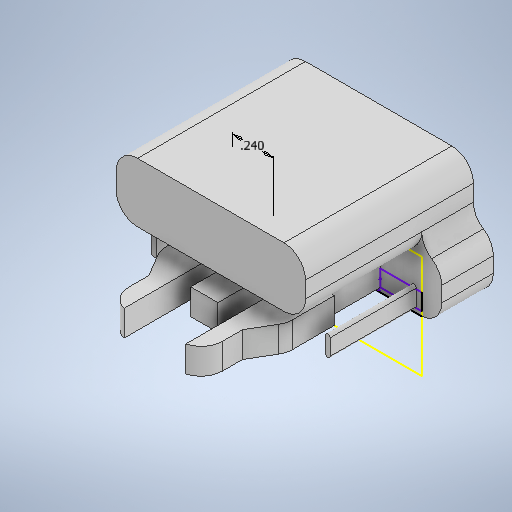
# Autodesk Inventor part: Attachment9
Saved by Autodesk Inventor 2025 (Build 290162010, 162A)
## iProperties
Created: 2026-02-26
Part Number: Attachment9
Material: Generic
Document SubType Name: Modeling
Designer: 925699
Density: 1 g/cm^3
Appearance: Default
Author: 925699
Autodesk Inventor part; units mm, degrees
ref_plane "YZ Plane" through (0, 0, 0) normal (1, 0, 0) x (0, 1, 0)
ref_plane "XZ Plane" through (0, 0, 0) normal (0, 1, 0) x (-1, 0, 0)
ref_plane "XY Plane" through (0, 0, 0) normal (0, 0, 1) x (1, 0, 0)
sketch "Sketch1" plane through (0, 0, 0) normal (0, 0, 1) x (1, 0, 0)
  line L0 (-6.3366, 6.9163) -> (21.6034, 6.9163)
  line L1 (21.6034, 6.9163) -> (21.6034, -8.3237)
  line L2 (21.6034, -8.3237) -> (-6.3366, -8.3237)
  line L3 (-6.3366, -8.3237) -> (-6.3366, 6.9163)
  point P0 (0, 0)
  dimension "d0" = 27.94
  dimension "d1" = 15.24
  constraints: 8 end point, 2 parallel, 1 horizontal, 1 perpendicular
  measures "d0" distance of L1.end L2.end
  measures "d1" distance of L0.end L1.end
extrude "Extrusion1" add sketch "Sketch1" along normal blind 7.62
sketch "Sketch2" plane through (0, 0, 7.62) normal (0, 0, 1) x (1, 0, 0)
  line L0 (-6.3366, 6.9163) -> (-6.3366, -8.3237) projected
  line L1 (21.6034, -8.3237) -> (21.6034, 6.9163) projected
  line L2 (21.6034, -0.052) -> (21.6034, 2.361)
  line L3 (-6.3366, 2.361) -> (-6.3366, -0.052)
  line L4 (21.6034, 6.9163) -> (-6.3366, 6.9163) projected
  line L5 (-6.3366, -8.3237) -> (21.6034, -8.3237) projected
  line L6 (0.9631, 2.361) -> (-0.2406, 2.361)
  line L7 (-0.2406, -0.052) -> (0.9631, -0.052)
  line L8 (-0.2406, -0.052) -> (-0.2406, 2.361)
  line L9 (-0.2406, -0.052) -> (3.0821, -0.052)
  line L10 (3.0821, -0.052) -> (3.0821, 2.361)
  line L11 (3.0821, 2.361) -> (-0.2406, 2.361)
  line L12 (-0.2406, 2.361) -> (-0.2406, -0.052)
  line L13 (14.3038, 2.361) -> (15.5074, 2.361)
  line L14 (15.5074, -0.052) -> (14.3038, -0.052)
  line L15 (15.5074, -0.052) -> (15.5074, 2.361)
  line L16 (15.5074, -0.052) -> (12.1847, -0.052)
  line L17 (12.1847, -0.052) -> (12.1847, 2.361)
  line L18 (12.1847, 2.361) -> (15.5074, 2.361)
  line L19 (15.5074, 2.361) -> (15.5074, -0.052)
  line L20 (-6.3366, -0.7037) -> (21.6034, -0.7037)
  line L21 (-6.3366, 2.361) -> (21.6034, 2.361)
  line L22 (21.6034, 2.361) -> (21.6034, -0.052)
  line L23 (21.6034, -0.052) -> (-6.3366, -0.052)
  line L24 (-6.3366, -0.052) -> (-6.3366, 2.361)
  point P0 (0, 0)
  point P1 (-0.2406, 1.1545)
  point P2 (15.2669, -0.3643)
  point P3 (15.5074, 1.1545)
  point P4 (15.5074, -0.052)
  point P5 (21.6034, -0.052)
  point P6 (15.5074, 2.361)
  point P7 (-6.3366, -0.052)
  point P8 (-0.2406, -0.052)
  point P9 (-0.2406, 2.361)
  point P10 (-6.3366, 2.361)
  point P11 (3.0821, -0.052)
  point P12 (12.1847, -0.052)
  point P13 (12.1847, 2.361)
  point P14 (3.0821, 2.361)
  dimension "d6" = 6.096
  constraints: 42 end point, 6 parallel, 4 perpendicular, 3 horizontal, 3 midpoint, 2 point on line
  measures "d6" distance from line of point (-0.241, 1.155) L0
extrude "Extrusion2" add sketch "Sketch2" along normal blind 8.7376 contours L6 L11 L10 L9 L7 L8 | L15 L14 L16 L17 L18 L13
sketch "Sketch3" plane through (-0.2406, 2.361, 7.62) normal (0, 1, 0) x (1, 0, 0)
  line L0 (3.3227, -8.7376) -> (0, -8.7376) projected
  line L1 (-6.096, 7.62) -> (21.844, 7.62) projected
  line L2 (3.3227, -11.3552) -> (3.3227, -8.7376)
  line L3 (12.4253, -11.3552) -> (12.4253, -8.7376)
  line L4 (17.2091, -8.255) -> (17.2091, -15.2732)
  line L5 (17.2091, -15.2732) -> (14.9854, -19.057)
  line L6 (14.9854, -19.057) -> (12.4253, -19.057)
  line L7 (12.4253, -19.057) -> (12.4253, -8.7376)
  line L8 (7.874, 7.62) -> (7.874, -24.8322)
  line L9 (3.3227, -11.3552) -> (3.3227, -8.7376)
  line L10 (-1.4611, -8.255) -> (-1.4611, -15.2732)
  line L11 (-1.4611, -15.2732) -> (0.7626, -19.057)
  line L12 (0.7626, -19.057) -> (3.3227, -19.057)
  line L13 (3.3227, -19.057) -> (3.3227, -8.7376)
  line L14 (17.2091, -8.255) -> (12.4253, -8.255)
  line L15 (12.4253, 0) -> (12.4253, -8.7376) projected
  line L16 (12.4253, -8.255) -> (12.4253, -8.7376)
  line L17 (-1.4611, -8.255) -> (3.3227, -8.255)
  line L18 (3.3227, 0) -> (3.3227, -8.7376) projected
  line L19 (3.3227, -8.255) -> (3.3227, -8.7376)
  point P0 (0.2406, 7.62)
  constraints: 32 end point, 4 perpendicular, 4 symmetric about line, 3 vertical, 1 collinear, 1 horizontal, 1 midpoint, 1 point on line
extrude "Extrusion4" add sketch "Sketch2" along normal blind 25.4 contours L6 L11 L10 L9 L7 L8 | L15 L14 L16 L17 L18 L13
sketch "Sketch4" plane through (-6.3366, 6.9163, 0) normal (0, 1, 0) x (1, 0, 0)
  point P0 (6.3366, 0)
sketch "Sketch5" plane through (0, 0, 7.62) normal (0, 0, 1) x (1, 0, 0)
  line L0 (21.6034, 6.9163) -> (-6.3366, 6.9163) projected
  line L1 (-6.3366, 15.6735) -> (21.6034, 15.6735)
  line L2 (21.6034, 15.6735) -> (21.6034, 6.9163)
  line L3 (21.6034, 6.9163) -> (-6.3366, 6.9163)
  line L4 (-6.3366, 6.9163) -> (-6.3366, 15.6735)
  point P0 (0, 0)
  constraints: 8 end point, 2 parallel, 1 horizontal, 1 perpendicular
extrude "Extrusion5" add sketch "Sketch5" along normal blind 17.145 and the other way blind 7.62
extrude "Extrusion6" cut sketch "Sketch2" against normal blind 25.4 contours L20 L1 L5 L0
extrude "Extrusion7" add sketch "Sketch2" along normal blind 4.7625 contours L21 L8 L23 L0 | L1 L23 L15 L21 | L21 L17 L23 L10
extrude "Extrusion8" add sketch "Sketch3" against normal up to surface (2.413 mm away)
sketch "Sketch6" plane through (-6.3366, -0.052, 7.62) normal (0, -1, 0) x (1, 0, 0)
  line L0 (27.94, 0) -> (27.94, 4.7625) projected
  line L1 (21.844, 4.7625) -> (21.844, 8.255) projected
  line L2 (27.94, 0) -> (21.844, 0)
  line L3 (21.844, 0) -> (21.844, 4.7625)
  line L4 (21.844, 4.7625) -> (27.94, 4.7625)
  line L5 (27.94, 4.7625) -> (27.94, 0)
  line L6 (18.5213, 4.7625) -> (18.5213, 25.4) projected
  line L7 (18.5213, 4.7625) -> (9.4187, 4.7625)
  line L8 (9.4187, 4.7625) -> (9.4187, 0)
  line L9 (9.4187, 0) -> (18.5213, 0)
  line L10 (18.5213, 0) -> (18.5213, 4.7625)
  line L11 (6.096, 4.7625) -> (6.096, 8.255) projected
  line L12 (0, 0) -> (0, 4.7625) projected
  line L13 (6.096, 4.7625) -> (0, 4.7625)
  line L14 (0, 4.7625) -> (0, 0)
  line L15 (0, 0) -> (6.096, 0)
  line L16 (6.096, 0) -> (6.096, 4.7625)
  point P0 (6.3366, -7.62)
  point P1 (21.844, 8.7376)
  point P2 (18.5213, 19.057)
  point P3 (6.096, 8.7376)
  constraints: 24 end point, 6 parallel, 3 horizontal, 3 perpendicular, 1 point on line
extrude "Extrusion9" cut sketch "Sketch6" against normal up to surface (6.9683 mm away)
sketch "Sketch7" plane through (12.1847, -0.052, 7.62) normal (0, -1, 0) x (1, 0, 0)
  line L0 (3.3227, 17.7594) -> (4.7838, 15.2732) projected
  line L1 (3.3227, 17.7594) -> (2.3659, 19.3874)
  line L2 (2.3659, 19.3874) -> (2.3659, 25.4)
  line L3 (3.3227, 25.4) -> (0, 25.4) projected
  line L4 (3.3227, 17.7594) -> (3.3227, 25.4) projected
  line L5 (2.3659, 25.4) -> (3.3227, 25.4)
  line L6 (3.3227, 25.4) -> (3.3227, 17.7594)
  line L7 (-18.5213, -7.62) -> (9.4187, -7.62) projected
  line L8 (-12.4253, 17.7594) -> (-11.4685, 19.3874)
  line L9 (-11.4685, 19.3874) -> (-11.4685, 25.4)
  line L10 (-12.4253, 17.7594) -> (-12.4253, 25.4)
  line L11 (-11.4685, 25.4) -> (-12.4253, 25.4)
  line L12 (-12.4253, 25.4) -> (-12.4253, 17.7594)
  line L13 (-12.4253, 8.7376) -> (-13.8865, 8.255) projected
  line L14 (-9.1825, 8.7376) -> (-9.1026, 8.7376)
  line L15 (-9.1026, 0) -> (-9.1026, 25.4) projected
  line L16 (-10.6842, 5.3569) -> (-10.764, 0)
  line L17 (-9.1026, 0) -> (-12.4253, 0) projected
  line L18 (-9.1026, 0) -> (-9.1026, 8.7376)
  line L19 (-10.764, 0) -> (-9.1026, 0)
  line L20 (9.4187, -7.62) -> (-18.5213, -7.62) projected
  line L21 (-18.5213, 17.145) -> (9.4187, 17.145) projected
  line L22 (1.5816, 5.3569) -> (1.6613, 0)
  line L23 (1.6613, 0) -> (0, 0)
  line L24 (0, 0) -> (0, 8.7376)
  line L25 (-4.5513, -7.62) -> (-4.5513, 0)
  line L26 (-4.5513, 11.274) -> (-4.5513, 11.3382)
  line L27 (-9.1026, 8.7376) -> (-10.6842, 5.3569)
  line L28 (0, 8.7376) -> (1.5816, 5.3569)
  point P0 (-12.1847, -7.62)
  constraints: 40 end point, 6 point on line, 4 collinear, 2 midpoint, 2 perpendicular, 1 horizontal, 1 vertical
extrude "Extrusion10" cut sketch "Sketch7" against normal up to surface (6.9683 mm away)
fillet "Fillet1" radius 3.175 4 edges at (0.7162, 1.1545, 33.02) (14.5507, 1.1545, 33.02) (16.9686, 1.1545, 22.8932) (-1.7017, 1.1545, 22.8932)
sketch "Sketch8" plane through (-0.2406, -0.052, 7.62) normal (0, -1, 0) x (1, 0, 0)
  arc A0 (-1.0234, 16.018) -> (-1.4611, 14.4093) centre (1.7139, 14.4093) ccw projected
  line L0 (-1.4611, 8.255) -> (-1.4611, 14.4093) projected
  line L1 (0, 0) -> (0, 8.255) projected
  line L2 (1.6613, 0) -> (0, 0) projected
  line L3 (1.6613, 0) -> (1.7411, 5.3569) projected
  line L4 (1.7411, 5.3569) -> (3.3227, 8.7376) projected
  line L5 (3.3227, 8.7376) -> (3.3227, 25.4) projected
  arc A1 (3.3227, 25.4) -> (0.9568, 22.3298) centre (4.1318, 22.3298) ccw projected
  line L6 (0.9568, 22.3298) -> (0.9568, 19.3874) projected
  line L7 (0.9568, 19.3874) -> (-1.0234, 16.018) projected
  arc A2 (17.2091, 14.4093) -> (16.7714, 16.018) centre (14.0341, 14.4093) ccw projected
  line L8 (16.7714, 16.018) -> (14.7912, 19.3874) projected
  line L9 (14.7912, 19.3874) -> (14.7912, 22.3298) projected
  arc A3 (14.7912, 22.3298) -> (12.4253, 25.4) centre (11.6162, 22.3298) ccw projected
  line L10 (12.4253, 8.7376) -> (12.4253, 25.4) projected
  line L11 (12.4253, 8.7376) -> (14.0069, 5.3569) projected
  line L12 (14.0069, 5.3569) -> (14.0867, 0) projected
  line L13 (15.748, 0) -> (14.0867, 0) projected
  line L14 (15.748, 0) -> (15.748, 8.255) projected
  line L15 (17.2091, 14.4093) -> (17.2091, 8.255) projected
  line L16 (17.2091, 8.255) -> (15.748, 8.255) projected
  line L17 (0, 8.255) -> (-1.4611, 8.255) projected
  point P0 (0.2406, -7.62)
extrude "Extrusion11" add sketch "Sketch8" against normal blind 3.81
sketch "Sketch9" plane through (0, 0, 7.62) normal (0, 0, 1) x (1, 0, 0)
  line L0 (9.6447, 0.3123) -> (5.6221, 0.3123)
  line L1 (5.6221, 0.3123) -> (5.6221, 4.1223)
  line L2 (5.6221, 4.1223) -> (9.6447, 4.1223)
  line L3 (9.6447, 4.1223) -> (9.6447, 0.3123)
  line L4 (12.1847, -0.052) -> (12.1847, 3.758) projected
  line L5 (3.0821, -0.052) -> (3.0821, 3.758) projected
  point P0 (0, 0)
  dimension "d30" = 2.54
  dimension "d31" = 2.54
  constraints: 8 end point, 2 parallel, 1 horizontal, 1 perpendicular
  measures "d30" distance between parallel lines of L4 L3
  measures "d31" distance between parallel lines of L1 L5
extrude "Extrusion12" add sketch "Sketch9" along normal blind 18.0975
sketch "Sketch10" plane through (21.6034, 6.9163, 24.765) normal (1, 0, 0) x (0, 0, -1)
  line L0 (17.145, 0) -> (0, 0) projected
  line L1 (24.765, -7.62) -> (17.145, -7.62) projected
  line L2 (17.145, 0) -> (24.765, 0)
  line L3 (24.765, 0) -> (24.765, -7.62)
  line L4 (24.765, -7.62) -> (17.145, -7.62)
  line L5 (17.145, -7.62) -> (17.145, 0)
  point P0 (24.765, -6.9163)
  constraints: 8 end point, 2 parallel, 1 horizontal, 1 perpendicular
extrude "Extrusion13" add sketch "Sketch10" along normal blind 2.9464 and the other way blind 34.0614
sketch "Sketch12" plane through (0, 0, 7.62) normal (0, 0, 1) x (1, 0, 0)
  line L0 (15.5074, 2.361) -> (15.5074, -0.052) projected
  line L1 (20.4604, -0.1957) -> (20.4604, 2.8523) construction
  line L2 (20.8033, 0.1472) -> (20.8033, 2.5094)
  line L3 (20.1175, 2.5094) -> (20.1175, 0.1472)
  arc A0 (20.1175, 0.1472) -> (20.8033, 0.1472) centre (20.4604, 0.1472) ccw
  arc A1 (20.8033, 2.5094) -> (20.1175, 2.5094) centre (20.4604, 2.5094) ccw
  line L4 (-12.458, -0.7037) -> (24.5498, -0.7037) projected
  line L5 (21.6034, 6.9163) -> (24.5498, 6.9163) projected
  line L6 (21.6034, 15.6735) -> (-6.3366, 15.6735) projected
  line L7 (7.6334, 15.6735) -> (7.6334, 10.1041)
  line L8 (-5.1936, -0.1957) -> (-5.1936, 2.8523) construction
  line L9 (-5.5365, 0.1472) -> (-5.5365, 2.5094)
  line L10 (-4.8507, 2.5094) -> (-4.8507, 0.1472)
  arc A2 (-5.5365, 0.1472) -> (-4.8507, 0.1472) centre (-5.1936, 0.1472) ccw
  arc A3 (-4.8507, 2.5094) -> (-5.5365, 2.5094) centre (-5.1936, 2.5094) ccw
  line L11 (6.0459, -0.7037) -> (6.0459, 5.9995)
  point P0 (0, 0)
  point P1 (20.4604, 1.3283)
  point P2 (20.4604, -0.1957)
  point P3 (20.4604, 2.8523)
  point P4 (-5.1936, 1.3283)
  point P5 (-5.1936, -0.1957)
  point P6 (-5.1936, 2.8523)
  dimension "d49" = 14.7574
  dimension "d50" = 14.0716
  dimension "d51" = 4.064
  dimension "d52" = 3.048
  constraints: 20 end point, 14 point on circle, 11 symmetric about line, 4 centre point, 4 point on line, 4 tangent, 3 midpoint, 3 vertical, 1 parallel, 2 other
  measures "d49" distance between parallel lines of L2 L11
  measures "d50" distance between parallel lines of L3 L11
  measures "d51" distance from line of L1.end L5
  measures "d52" distance of L1.end L1.start
extrude "Extrusion16" add sketch "Sketch12" along normal blind 12.7
fillet "Fillet2" radius 3.175 10 edges at (-12.458, 6.9163, 3.81) (-12.458, -0.7037, 3.81) (24.5498, -0.7037, 3.81) (24.5498, 6.9163, 3.81) (21.6034, 6.9163, 3.81) (-6.3366, 6.9163, 3.81) (-6.3366, 15.6735, 12.3825) (21.6034, 15.6735, 12.3825) (21.6034, 6.9163, 16.1925) (-6.3366, 6.9163, 16.1925)
body "Solid1"
